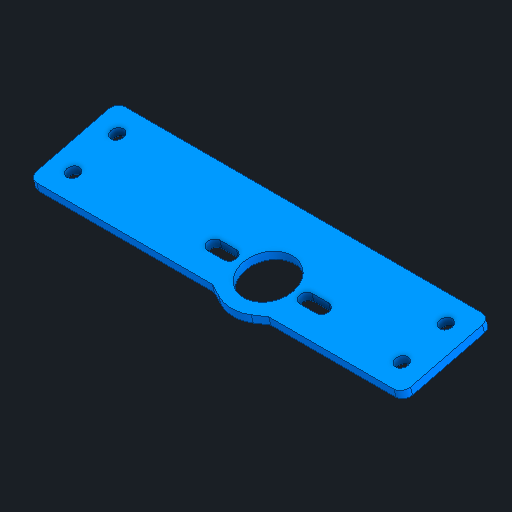
# Autodesk Inventor part: motor_mount_plate
Saved by Autodesk Inventor 2023 (Build 270158030, 158C)
## iProperties
Created: 2022-03-30
Part Number: motor_mount_plate
Material: Generic
Document SubType Name: Modeling
Designer: kardo
Density: 1 g/cm^3
Appearance: Blue Plastic
Author: kardo
Autodesk Inventor part; units mm, degrees
ref_plane "YZ Plane" through (0, 0, 0) normal (1, 0, 0) x (0, 1, 0)
ref_plane "XZ Plane" through (0, 0, 0) normal (0, 1, 0) x (-1, 0, 0)
ref_plane "XY Plane" through (0, 0, 0) normal (0, 0, 1) x (1, 0, 0)
derived "stencil_frame.ipt"
sketch "sk_cowl_joint_locations" plane through (54.6, 0, 0) normal (1, 0, 0) x (0, 1, 0)
  line L0 (-345, 16.32) -> (-262.2001, 18.586) construction
  arc A0 (-262.2001, 18.586) -> (-241.5001, 19.2432) centre (-326.8578, 2381.2399) ccw construction
  line L1 (-241.5001, 19.2432) -> (11.22, 28.376) construction
  arc A1 (36.465, 28.832) -> (11.22, 28.376) centre (36.465, -670.197) ccw construction
  line L2 (36.465, 28.832) -> (112.2, 28.832) construction
  line L3 (94.8, 30.032) -> (36.465, 30.032) construction
  arc A2 (36.465, 30.032) -> (11.1767, 29.5752) centre (36.465, -670.197) ccw construction
  line L4 (11.1767, 29.5752) -> (-241.5434, 20.4424) construction
  arc A3 (-262.2329, 19.7855) -> (-241.5434, 20.4424) centre (-326.8578, 2381.2399) ccw construction
  line L5 (-262.2329, 19.7855) -> (-345, 17.5204) construction
  line L6 (-230.0001, 3089.1136) -> (-230.0001, -1866.0023) construction
  line L7 (-114.9999, 3089.1136) -> (-114.9999, -1866.0023) construction
  line L8 (-345, 3089.1136) -> (-345, -1866.0023) construction
  line L9 (0, 3089.1136) -> (0, -1866.0023) construction
  line L10 (-230.0001, 45.0685) -> (-230.0001, 20.8596) construction
  line L11 (-114.9999, 49.9659) -> (-114.9999, 25.0155) construction
  line L12 (-345, 17.5204) -> (-345, 17.5204)
  line L13 (-345, 17.5204) -> (-345, 36.9221) construction
  line L14 (-869.78, 3004.1953) -> (348.339, -1881.413) construction
  line L15 (-344.7623, 36.9221) -> (-345, 39.712) construction
  line L16 (0, 51.6) -> (0, 29.1713) construction
  line L17 (-136.2088, 45.4676) -> (-130.9657, 24.4385) construction
  line L18 (-128.3953, 30.6635) -> (-132.2764, 29.6958) construction
  line L19 (-131.0168, 41.178) -> (-134.898, 40.2103) construction
  line L20 (-136.2088, 45.4676) -> (-132.3276, 46.4353) construction
  line L21 (-130.9657, 24.4385) -> (-127.0845, 25.4062) construction
  line L22 (-132.3276, 46.4353) -> (-132.5171, 52.2322) construction
  spline S0 degree 2 poles (-345, 39.712) (-172.656, 54.3934) (0, 54.4) knots 0 0 0 1 1 1
  spline S1 degree 3 poles (0, 54.4) (37.026, 54.4) (80.784, 47.9917) (112.2, 37.536) knots 1 1 1 1 2 2 2 2
  spline S2 degree 3 poles (111.3158, 34.8793) (106.1488, 36.5989) (96.4909, 39.4217) (84.5445, 42.2265) (75.2974, 44.1359) (69.0059, 45.3094) (61.0256, 46.6466) (54.5653, 47.6105) (46.4371, 48.6777) (39.9092, 49.4192) (31.7597, 50.2005) (25.2653, 50.7072) (17.2211, 51.1873) (9.2717, 51.5118) (3.0586, 51.6) (0, 51.6) knots 1 1 1 1 1.166667 1.291667 1.333333 1.416667 1.458333 1.541667 1.583333 1.666667 1.708333 1.791667 1.833333 1.916667 2 2 2 2
  spline S3 degree 3 poles (0, 51.6) (-19.1708, 51.5993) (-52.7146, 51.3604) (-91.0402, 50.6121) (-119.7801, 49.8472) (-138.9379, 49.2354) (-162.8824, 48.3434) (-182.0358, 47.528) (-205.975, 46.3814) (-225.1241, 45.3623) (-249.0578, 43.9611) (-268.2026, 42.7383) (-292.131, 41.0825) (-316.0566, 39.2994) (-335.1942, 37.7372) (-344.7623, 36.9221) knots 0 0 0 0 0.166667 0.291667 0.333333 0.416667 0.458333 0.541666 0.583333 0.666666 0.708333 0.791666 0.833333 0.916666 1 1 1 1
  point P0 (0, 0)
  point P1 (-345, 27.2213)
  point P2 (-230.0001, 32.964)
  point P3 (-114.9999, 37.4907)
  point P4 (0, 40.3857)
  point P5 (0, 40.3857)
ref_plane "plane_motor_mount" through (0, -120.75, 0) normal (0, 0.9702957, 0.2419219) x (-1, 0, 0)
ref_plane "plane_symmetry" through (0, 0, 0) normal (1, 0, 0) x (0, 1, 0)
sketch "sk_drivetrain_profile" plane through (6, 0, 0) normal (1, 0, 0) x (0, 1, 0)
  line L0 (-529.1913, 0) -> (410.1479, 0) construction
  line L1 (-345, 3089.1136) -> (-345, -1866.0023) construction
  line L2 (0, 3089.1136) -> (0, -1866.0023) construction
  line L3 (-134.0777, 53.4546) -> (-127.3039, 26.2863)
  line L4 (-377, 0) -> (-313.1194, 3.9071)
  line L5 (-130.6908, 39.8704) -> (-224.6958, 16.4323)
  line L6 (-301.4275, 4.6222) -> (-262.5191, 7.002) construction
  line L7 (-262.5191, 7.002) -> (-224.6958, 16.4323) construction
  line L8 (-127.3039, 26.2863) -> (-127.3039, 21.2863) construction
  line L9 (-313.1194, 3.9071) -> (-301.4275, 4.6222)
  line L10 (-869.78, 3004.1953) -> (348.339, -1881.413) construction
  line L11 (-225.3679, 19.1279) -> (-131.3629, 42.566) construction
  line L12 (-130.0187, 37.1748) -> (-224.0238, 13.7367) construction
  line L13 (-225.3679, 19.1279) -> (-224.0238, 13.7367) construction
  spline S0 degree 2 poles (-301.4275, 4.6222) (-262.5191, 7.002) (-224.6958, 16.4323) knots 1 1 1 2 2 2
  line L14 (0, 21.3303) -> (-241.5001, 18.9703) construction
  line L15 (-49.1478, 22.05) -> (-303.2844, 19.5666) construction
  point P0 (0, 0)
  point P1 (-213.4159, 19.2447)
  point P2 (-201.4639, 19.3615)
  point P3 (-196.4544, 20.6106)
derived "parameters_frame.ipt"
sketch "sk_base" plane through (0, -120.75, 0) normal (0, 0.9702957, 0.2419219) x (-1, 0, 0)
  line L0 (0, -1322.9835) -> (0, 2988.4132) projected
  line L1 (-44.6, 47.8569) -> (-44.6, 26.1839)
  line L2 (-44.6, 26.1839) -> (0, 26.1839)
  line L3 (-44.6, 47.8569) -> (0, 47.8569)
  point P0 (0, -29.2121)
  point P1 (-54.6, 47.8569)
  point P2 (-54.6, 26.1839)
  dimension "d1" = 10
  constraints: 6 end point, 4 point on line, 2 perpendicular, 1 parallel
  measures "d1" distance from line of point (-54.6, 47.857) L1
extrude "base" add sketch "sk_base" against normal blind 2
sketch "sk_drill_joint" plane through (0, -120.75, 0) normal (0, 0.9702957, 0.2419219) x (-1, 0, 0)
  line L0 (-44.6, 47.8569) -> (-44.6, 26.1839) construction
  line L1 (-44.6, 47.8569) -> (0, 47.8569) construction
  line L2 (-44.6, 26.1839) -> (0, 26.1839) construction
  circle A0 centre (-39.2, 31.5839) radius 1.5
  circle A1 centre (-39.2, 42.4569) radius 1.5
  line L3 (-39.2, 42.4569) -> (-39.2, 47.8569) construction
  line L4 (-39.2, 42.4569) -> (-39.2, 31.5839) construction
  line L5 (-39.2, 31.5839) -> (-39.2, 26.1839) construction
  line L6 (-39.2, 42.4569) -> (-44.6, 42.4569) construction
  line L7 (-39.2, 31.5839) -> (-44.6, 31.5839) construction
  point P0 (0, -29.2121)
  dimension "d3" = 3
  dimension "d4" = 5.4
  constraints: 10 end point, 4 perpendicular, 4 point on line, 2 centre point, 2 collinear, 1 coincident, 1 equal radius, 1 parallel
  measures "d3" diameter of A1
  measures "d4" distance between parallel lines of L0 L4
extrude "drill_joint" cut sketch "sk_drill_joint" along normal through all both and the other way through all
mirror "mirror" about plane through (0, 0, 0) normal (1, 0, 0)
sketch "sk_expand_motor" plane through (0, -120.75, 0) normal (0, 0.9702957, 0.2419219) x (-1, 0, 0)
  line L0 (-6, 55.091) -> (-6, 27.091) construction
  line L1 (-9.8571, 49.2226) -> (-21.2857, 43.8015)
  arc A0 (-21.2857, 43.8015) -> (-21.2857, 38.3805) centre (-20, 41.091) ccw
  line L2 (-21.2857, 38.3805) -> (-9.8571, 32.9594)
  arc A1 (-9.8571, 32.9594) -> (-2.1429, 32.9594) centre (-6, 41.091) ccw
  line L3 (-2.1429, 32.9594) -> (9.2857, 38.3805)
  arc A2 (9.2857, 38.3805) -> (9.2857, 43.8015) centre (8, 41.091) ccw
  line L4 (9.2857, 43.8015) -> (-2.1429, 49.2226)
  arc A3 (-2.1429, 49.2226) -> (-9.8571, 49.2226) centre (-6, 41.091) ccw
  line L5 (-20, 41.091) -> (8, 41.091) construction
  point P0 (0, -29.2121)
  dimension "d23" = 28
  dimension "d24" = 18
  dimension "d26" = 6
  constraints: 10 end point, 8 point on circle, 8 tangent, 4 centre point, 3 midpoint, 2 coincident, 2 equal radius, 1 perpendicular
  measures "d23" distance of L5.end L5.start
  measures "d24" diameter of A3
  measures "d26" diameter of A2
extrude "expand_motor" add sketch "sk_expand_motor" against normal blind 2
sketch "sk_drill_motor" plane through (0, -120.75, 0) normal (0, 0.9702957, 0.2419219) x (-1, 0, 0)
  circle A0 centre (-6, 41.091) radius 6
  line L0 (-15, 41.091) -> (-19, 41.091) construction
  line L1 (-15, 42.591) -> (-19, 42.591)
  line L2 (-19, 39.591) -> (-15, 39.591)
  arc A1 (-15, 39.591) -> (-15, 42.591) centre (-15, 41.091) ccw
  arc A2 (-19, 42.591) -> (-19, 39.591) centre (-19, 41.091) ccw
  line L3 (3, 41.091) -> (7, 41.091) construction
  line L4 (3, 39.591) -> (7, 39.591)
  line L5 (7, 42.591) -> (3, 42.591)
  arc A3 (3, 42.591) -> (3, 39.591) centre (3, 41.091) ccw
  arc A4 (7, 39.591) -> (7, 42.591) centre (7, 41.091) ccw
  line L6 (-15, 41.091) -> (-6, 41.091) construction
  line L7 (-6, 41.091) -> (3, 41.091) construction
  line L8 (-6, 55.091) -> (-6, 27.091) construction
  point P0 (0, -29.2121)
  point P1 (-17, 41.091)
  point P2 (5, 41.091)
  dimension "d9" = 12
  dimension "d14" = 3
  dimension "d15" = 4
  dimension "d21" = 18
  constraints: 20 end point, 8 point on circle, 8 tangent, 5 centre point, 5 collinear, 2 midpoint, 2 parallel, 1 equal radius, 1 perpendicular
  measures "d9" diameter of A0
  measures "d14" diameter of A2
  measures "d15" distance of L2.start L2.end
  measures "d21" distance of L3.start L0.start
extrude "drill_motor" cut sketch "sk_drill_motor" along normal through all both and the other way through all
fillet "round_corners" radius 2 4 edges at (44.6, -133.2979, 46.1934) (44.6, -128.0548, 25.1642) (-44.6, -133.2979, 46.1934) (-44.6, -128.0548, 25.1642)
derived "parameters_powertrain.ipt"
equation "\"d1\" = cowl_sealing_width + cowl_liner_width"
equation "\"d3\" = drill_motor_mount_diam"
equation "\"d4\" = 1.8 * drill_motor_mount_diam"
equation "\"d27\" = bulkhead_thickness"
equation "\"d18\" = 0.5 * bulkhead_inset"
equation "\"drill_motor_mount_diam\" = 3"
equation "\"bulkhead_thickness\" = 2"
equation "\"bulkhead_inset\" = 4"
equation "\"cowl_sealing_width\" = 5"
equation "\"cowl_liner_width\" = 5"
body "Solid1"
